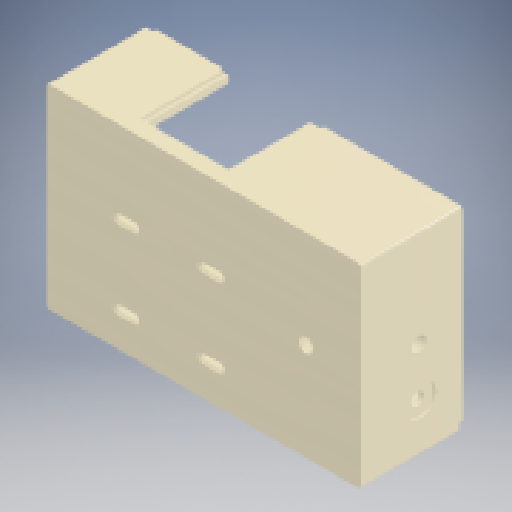
# Autodesk Inventor part: First_Stage_BoxBottom_Print
Saved by Autodesk Inventor 2025.2 (Build 292293000, 293)
## iProperties
Created: 2024-12-04
Part Number: First_Stage_BoxBottom_Print
Material: Generic
Document SubType Name: Modeling
Designer: Paul Linke
Density: 1 g/cm^3
Appearance: Light Beige
Author: Paul Linke
Autodesk Inventor part; units mm, degrees
ref_plane "YZ Plane" through (0, 0, 0) normal (1, 0, 0) x (0, 1, 0)
ref_plane "XZ Plane" through (0, 0, 0) normal (0, 1, 0) x (-1, 0, 0)
ref_plane "XY Plane" through (0, 0, 0) normal (0, 0, 1) x (1, 0, 0)
sketch "Sketch1" plane through (0, 0, 0) normal (0, 0, 1) x (1, 0, 0)
  line L0 (132.8531, -39.939) -> (132.8531, -33.679) projected
  line L1 (-45.1505, -5.78) -> (-45.1505, -12.04) projected
  circle A0 centre (47.6, -44.5) radius 1.45 projected
  circle A1 centre (0, -44.5) radius 1.45 projected
  circle A2 centre (0, 0) radius 1.45 projected
  circle A3 centre (47.5, 0) radius 1.45 projected
  line L2 (132.8531, -63.939) -> (-45.1505, -63.939)
  line L3 (-45.1505, 46.119) -> (132.8531, 46.119)
  line L4 (132.8531, 46.119) -> (132.8531, -63.939)
  line L5 (-45.1505, -63.939) -> (-45.1505, -12.04)
  line L6 (-45.1505, 46.119) -> (-45.1505, -5.78)
  line L7 (-45.1505, -12.04) -> (-45.1505, -5.78)
  line L8 (52.6, -44.5) -> (42.6, -44.5) construction
  line L9 (52.6, -43.05) -> (42.6, -43.05)
  line L10 (42.6, -45.95) -> (52.6, -45.95)
  arc A4 (52.6, -45.95) -> (52.6, -43.05) centre (52.6, -44.5) ccw
  arc A5 (42.6, -43.05) -> (42.6, -45.95) centre (42.6, -44.5) ccw
  line L11 (5, -44.5) -> (-5, -44.5) construction
  line L12 (5, -43.05) -> (-5, -43.05)
  line L13 (-5, -45.95) -> (5, -45.95)
  arc A6 (5, -45.95) -> (5, -43.05) centre (5, -44.5) ccw
  arc A7 (-5, -43.05) -> (-5, -45.95) centre (-5, -44.5) ccw
  line L14 (5, 0) -> (-5, 0) construction
  line L15 (5, 1.45) -> (-5, 1.45)
  line L16 (-5, -1.45) -> (5, -1.45)
  arc A8 (5, -1.45) -> (5, 1.45) centre (5, 0) ccw
  arc A9 (-5, 1.45) -> (-5, -1.45) centre (-5, 0) ccw
  line L17 (52.5, 0) -> (42.5, 0) construction
  line L18 (52.5, 1.45) -> (42.5, 1.45)
  line L19 (42.5, -1.45) -> (52.5, -1.45)
  arc A10 (52.5, -1.45) -> (52.5, 1.45) centre (52.5, 0) ccw
  arc A11 (42.5, 1.45) -> (42.5, -1.45) centre (42.5, 0) ccw
  point P0 (0, 0)
  dimension "d1" = 24
  dimension "d2" = 10
  dimension "d3" = 10
  dimension "d4" = 10
  dimension "d5" = 10
  constraints: 44 end point, 20 tangent, 16 point on circle, 8 centre point, 8 equal length, 4 midpoint, 2 collinear, 2 horizontal, 2 point on line, 1 vertical
  measures "d1" distance from line of L0.start L2
  measures "d2" distance of L8.end L8.start
  measures "d3" distance of L11.end L11.start
  measures "d4" distance of L17.end L17.start
  measures "d5" distance of L14.end L14.start
extrude "Extrusion1" add sketch "Sketch1" along normal blind 5
sketch "Sketch2" plane through (0, 0, 0) normal (0, 0, -1) x (-1, 0, 0)
  line L0 (41.1505, -59.939) -> (-128.8531, -59.939)
  line L1 (-128.8531, -59.939) -> (-128.8531, 42.119)
  line L2 (-128.8531, 42.119) -> (41.1505, 42.119)
  line L3 (41.1505, 42.119) -> (41.1505, -59.939)
  line L4 (45.1505, -63.939) -> (-132.8531, -63.939) projected
  line L5 (45.1505, 46.119) -> (45.1505, -63.939) projected
  line L6 (-132.8531, 46.119) -> (45.1505, 46.119) projected
  line L7 (-132.8531, -63.939) -> (-132.8531, 46.119) projected
  point P0 (0, 0)
  dimension "d8" = 4
  dimension "d9" = 4
  dimension "d10" = 4
  dimension "d11" = 4
  constraints: 8 end point, 2 parallel, 1 horizontal, 1 perpendicular
  measures "d8" distance between parallel lines of L0 L4
  measures "d9" distance between parallel lines of L5 L3
  measures "d10" distance between parallel lines of L2 L6
  measures "d11" distance between parallel lines of L7 L1
extrude "Extrusion2" add sketch "Sketch2" along normal blind 50
fillet "Fillet1" radius 2 4 edges at (-45.1505, 46.119, -22.5) (132.8531, 46.119, -22.5) (-45.1505, -63.939, -22.5) (132.8531, -63.939, -22.5)
fillet "Fillet2" radius 15 4 edges at (128.8531, -59.939, -25) (-41.1505, -59.939, -25) (-41.1505, 42.119, -25) (128.8531, 42.119, -25)
sketch "Sketch5" plane through (0, 0, -50) normal (0, 0, -1) x (-1, 0, 0)
  arc A0 (-132.8531, -61.939) -> (-130.8531, -63.939) centre (-130.8531, -61.939) ccw projected
  line L0 (-130.8531, -63.939) -> (43.1505, -63.939) projected
  arc A1 (43.1505, -63.939) -> (45.1505, -61.939) centre (43.1505, -61.939) ccw projected
  line L1 (45.1505, -61.939) -> (45.1505, 44.119) projected
  arc A2 (45.1505, 44.119) -> (43.1505, 46.119) centre (43.1505, 44.119) ccw projected
  line L2 (43.1505, 46.119) -> (-130.8531, 46.119) projected
  arc A3 (-130.8531, 46.119) -> (-132.8531, 44.119) centre (-130.8531, 44.119) ccw projected
  line L3 (-132.8531, 44.119) -> (-132.8531, -61.939) projected
  line L4 (26.1505, -59.939) -> (-113.8531, -59.939) projected
  arc A4 (-128.8531, -44.939) -> (-113.8531, -59.939) centre (-113.8531, -44.939) ccw projected
  line L5 (-128.8531, -44.939) -> (-128.8531, 27.119) projected
  arc A5 (-113.8531, 42.119) -> (-128.8531, 27.119) centre (-113.8531, 27.119) ccw projected
  line L6 (-113.8531, 42.119) -> (26.1505, 42.119) projected
  arc A6 (41.1505, 27.119) -> (26.1505, 42.119) centre (26.1505, 27.119) ccw projected
  line L7 (41.1505, 27.119) -> (41.1505, -44.939) projected
  arc A7 (26.1505, -59.939) -> (41.1505, -44.939) centre (26.1505, -44.939) ccw projected
  line L8 (43.1505, -61.939) -> (-130.8531, -61.939)
  line L9 (-130.8531, -61.939) -> (-130.8531, 44.119)
  line L10 (-130.8531, 44.119) -> (43.1505, 44.119)
  line L11 (43.1505, 44.119) -> (43.1505, -61.939)
  point P0 (0, 0)
  constraints: 8 end point, 2 parallel, 1 horizontal, 1 perpendicular
extrude "Extrusion3" add sketch "Sketch5" along normal blind 4 contours L8 L9 L10 L11
fillet "Fillet3" radius 2 4 edges at (-43.1505, 44.119, -52) (130.8531, 44.119, -52) (130.8531, -61.939, -52) (-43.1505, -61.939, -52)
sketch "Sketch12" plane through (-43.1505, -63.939, 5) normal (0, -1, 0) x (1, 0, 0)
  line L0 (157.0036, -5) -> (17, -5) projected
  line L1 (17, -59) -> (157.0036, -59) projected
  line L2 (91.972, -5) -> (41.972, -5)
  line L3 (41.972, -5) -> (41.972, -59)
  line L4 (41.972, -59) -> (91.972, -59)
  line L5 (91.972, -59) -> (91.972, -5)
  line L6 (91.972, -59) -> (41.972, -59)
  line L7 (91.972, -5) -> (41.972, -5)
  line L8 (91.972, -9) -> (41.972, -9)
  line L9 (41.972, -9) -> (41.972, -5)
  line L10 (41.972, -5) -> (91.972, -5)
  line L11 (91.972, -5) -> (91.972, -9)
  line L12 (95.972, -5) -> (95.972, -59)
  line L13 (37.972, -59) -> (37.972, -5)
  point P0 (43.1505, -5)
  point P1 (84.472, -31.9556)
  point P2 (49.472, -31.9556)
  point P3 (91.972, -32)
  point P4 (41.972, -32)
  dimension "d41" = 7.5
  dimension "d42" = 7.5
  dimension "d49" = 4
  constraints: 24 end point, 5 equal length, 3 perpendicular, 3 point on line, 2 horizontal, 2 midpoint, 2 vertical, 6 other
  measures "d41" horizontal distance of point (91.972, -32) point (84.472, -31.956)
  measures "d42" horizontal distance of point (41.972, -32) point (49.472, -31.956)
  measures "d49" distance between parallel lines of L0 L8
extrude "Extrusion9" cut sketch "Sketch12" against normal blind 150 contours L5 L1 L3 L8
sketch "Sketch13" plane through (113.8531, -59.939, 0) normal (0, 1, 0) x (1, 0, 0)
  line L0 (-140.0036, 54) -> (-115.0316, 54) projected
  line L1 (0, 0) -> (-140.0036, 0) projected
  line L2 (-119.0316, 54) -> (-61.0316, 54)
  line L3 (-61.0316, 54) -> (-61.0316, 0)
  line L4 (-61.0316, 0) -> (-119.0316, 0)
  line L5 (-119.0316, 0) -> (-119.0316, 54)
  line L6 (-115.0316, 4) -> (-115.0316, 54) projected
  line L7 (-65.0316, 54) -> (-65.0316, 4) projected
  point P0 (-113.8531, 0)
  point P1 (-75.0316, 0)
  point P2 (-125.0316, 0)
  point P3 (-65.0316, 4)
  point P4 (-119.0316, 0)
  dimension "d45" = 4
  dimension "d46" = 4
  constraints: 8 end point, 2 parallel, 2 point on line, 1 horizontal, 1 perpendicular, 2 other
extrude "Extrusion10" cut sketch "Sketch13" along normal blind 104.0581 and the other way blind 2
sketch "Sketch15" plane through (113.8531, -59.939, 0) normal (0, 1, 0) x (1, 0, 0)
  line L0 (-61.0316, 50) -> (-61.0316, 54) projected
  line L1 (-61.0316, 50) -> (-61.0316, 0) projected
  line L2 (-61.0316, 0) -> (-119.0316, 0) projected
  line L3 (-119.0316, 0) -> (-119.0316, 50) projected
  line L4 (-119.0316, 54) -> (-119.0316, 50) projected
  line L5 (-114.9316, 4.1) -> (-114.9316, 50)
  line L6 (-115.0316, 50) -> (-115.0316, 4) projected
  line L7 (-115.0316, 4) -> (-65.0316, 4) projected
  line L8 (-65.0316, 4) -> (-65.0316, 50) projected
  line L9 (-65.0316, 50) -> (-65.0316, 4) projected
  line L10 (0, 0) -> (-61.0316, 0) projected
  line L11 (-65.0316, 50) -> (-57.0316, 50)
  line L12 (-57.0316, 50) -> (-57.0316, 0)
  line L13 (-57.0316, 0) -> (-65.0316, 0)
  line L14 (-65.0316, 0) -> (-65.0316, 50)
  line L15 (-115.0316, 50) -> (-123.0316, 50)
  line L16 (-123.0316, 50) -> (-123.0316, 0)
  line L17 (-123.0316, 0) -> (-115.0316, 0)
  line L18 (-115.0316, 0) -> (-115.0316, 50)
  line L19 (-65.0316, 4) -> (-115.0316, 4)
  line L20 (-115.0316, 4) -> (-115.0316, 0)
  line L21 (-115.0316, 0) -> (-65.0316, 0)
  line L22 (-65.0316, 0) -> (-65.0316, 4)
  line L23 (-57.0316, 50) -> (-65.0316, 50)
  line L24 (-65.0316, 50) -> (-65.0316, 54)
  line L25 (-65.0316, 54) -> (-57.0316, 54)
  line L26 (-57.0316, 54) -> (-57.0316, 50)
  line L27 (-115.0316, 50) -> (-119.0316, 50) projected
  line L28 (-140.0036, 54) -> (-119.0316, 54) projected
  line L29 (-115.0316, 50) -> (-123.0316, 50)
  line L30 (-123.0316, 50) -> (-123.0316, 54)
  line L31 (-123.0316, 54) -> (-115.0316, 54)
  line L32 (-115.0316, 54) -> (-115.0316, 50)
  point P0 (-119.0316, 0)
  dimension "d124" = 8
  dimension "d125" = 8
  constraints: 42 end point, 10 parallel, 5 horizontal, 5 perpendicular, 3 point on line, 1 vertical, 2 other
  measures "d124" distance of L12.end L13.end
  measures "d125" distance of L17.end L16.end
extrude "Extrusion12" add sketch "Sketch15" along normal blind 4
sketch "Sketch17" plane through (-45.1505, -61.939, 5) normal (-1, 0, 0) x (0, 0, 1)
  line L0 (-55, -2) -> (0, -2) projected
  line L1 (0, 108.058) -> (-55, 108.058) projected
  line L2 (0, 106.058) -> (-55, 106.058) projected
  circle A0 centre (-32.44, 53.029) radius 2.305
  circle A1 centre (-32.44, 53.029) radius 3.5
  point P0 (-5, 61.939)
  dimension "d114" = 7
  constraints: 2 centre point, 1 coincident, 2 other
  measures "d114" diameter of A1
extrude "Extrusion14" cut sketch "Sketch17" against normal blind 10 contours A0 | A1
sketch "Sketch18" plane through (-45.1505, -61.939, 5) normal (-1, 0, 0) x (0, 0, 1)
  circle A0 centre (-32.44, 53.029) radius 2.555
  circle A1 centre (-32.44, 53.029) radius 3.5 projected
  circle A2 centre (-32.44, 53.029) radius 9
  point P0 (-5, 61.939)
  dimension "d115" = 18
  constraints: 2 centre point, 1 coincident, 2 other
  measures "d115" diameter of A2
extrude "Extrusion15" cut sketch "Sketch18" against normal blind 1.3 contours A0 | A1 | A2
sketch "Sketch19" plane through (132.8531, -61.939, -50) normal (1, 0, 0) x (0, 0, -1)
  circle A0 centre (-21.8645, 25.1387) radius 2.425
  circle A1 centre (-21.8645, 25.1387) radius 3.5
  point P0 (-50, 61.939)
  dimension "d116" = 7
  constraints: 2 centre point, 1 coincident, 2 other
  measures "d116" diameter of A1
extrude "Extrusion16" cut sketch "Sketch19" against normal blind 10 contours A0 | A1
sketch "Sketch20" plane through (132.8531, -61.939, -50) normal (1, 0, 0) x (0, 0, -1)
  circle A0 centre (-21.8645, 25.1387) radius 2.555
  circle A1 centre (-21.8645, 25.1387) radius 9
  point P0 (-50, 61.939)
  dimension "d117" = 18
  constraints: 2 centre point, 1 coincident, 2 other
  measures "d117" diameter of A1
extrude "Extrusion17" cut sketch "Sketch20" against normal blind 1.3 contours A0 | A1
sketch "Sketch23" plane through (0, 0, 0) normal (0, 0, -1) x (-1, 0, 0)
  line L0 (9.1785, -59.939) -> (26.1505, -59.939) projected
  arc A0 (26.1505, -59.939) -> (41.1505, -44.939) centre (26.1505, -44.939) ccw projected
  line L1 (41.1505, -44.939) -> (41.1505, 27.119) projected
  arc A1 (41.1505, 27.119) -> (26.1505, 42.119) centre (26.1505, 27.119) ccw projected
  line L2 (26.1505, 42.119) -> (5.1785, 42.119) projected
  arc A2 (-113.8531, 42.119) -> (-128.8531, 27.119) centre (-113.8531, 27.119) ccw projected
  line L3 (-128.8531, 27.119) -> (-128.8531, -44.939) projected
  arc A3 (-128.8531, -44.939) -> (-113.8531, -59.939) centre (-113.8531, -44.939) ccw projected
  line L4 (-113.8531, -59.939) -> (-56.8215, -59.939) projected
  arc A4 (-52.6, -43.05) -> (-52.6, -45.95) centre (-52.6, -44.5) ccw projected
  line L5 (-42.6, -43.05) -> (-52.6, -43.05) projected
  arc A5 (-42.6, -45.95) -> (-42.6, -43.05) centre (-42.6, -44.5) ccw projected
  line L6 (-52.6, -45.95) -> (-42.6, -45.95) projected
  arc A6 (-5, -43.05) -> (-5, -45.95) centre (-5, -44.5) ccw projected
  line L7 (5, -43.05) -> (-5, -43.05) projected
  arc A7 (5, -45.95) -> (5, -43.05) centre (5, -44.5) ccw projected
  line L8 (-5, -45.95) -> (5, -45.95) projected
  arc A8 (-5, 1.45) -> (-5, -1.45) centre (-5, 0) ccw projected
  line L9 (5, 1.45) -> (-5, 1.45) projected
  arc A9 (5, -1.45) -> (5, 1.45) centre (5, 0) ccw projected
  line L10 (-5, -1.45) -> (5, -1.45) projected
  arc A10 (-52.5, 1.45) -> (-52.5, -1.45) centre (-52.5, 0) ccw projected
  line L11 (-42.5, 1.45) -> (-52.5, 1.45) projected
  arc A11 (-42.5, -1.45) -> (-42.5, 1.45) centre (-42.5, 0) ccw projected
  line L12 (-52.5, -1.45) -> (-42.5, -1.45) projected
  line L13 (-73.8531, 6.09) -> (-128.8531, 6.09)
  line L14 (-128.8531, 6.09) -> (-128.8531, -23.91)
  line L15 (-128.8531, -23.91) -> (-73.8531, -23.91)
  line L16 (-73.8531, -23.91) -> (-73.8531, 6.09)
  line L17 (-128.8531, -44.939) -> (-128.8531, 27.119) projected
  line L18 (43.1505, 46.119) -> (-130.8531, 46.119) projected
  line L19 (-107.0925, 46.119) -> (-107.0925, 6.09) construction
  line L20 (-106.4911, -23.91) -> (-106.4911, -63.939) construction
  line L21 (43.1505, -63.939) -> (-130.8531, -63.939) projected
  line L22 (5.1785, 44.1191) -> (5.1785, 42.119) projected
  line L23 (-52.8215, 42.119) -> (-52.8215, 44.1191) projected
  line L24 (-52.8215, -61.939) -> (5.1785, -61.939) projected
  line L25 (5.1785, 44.1191) -> (-52.8215, 44.1191) projected
  line L26 (-52.8215, 42.119) -> (-113.8531, 42.119) projected
  line L27 (-52.8215, -61.939) -> (-52.8215, -59.939) projected
  line L28 (5.1785, -59.939) -> (5.1785, -61.939) projected
  line L29 (-56.8215, -59.939) -> (-56.8215, -55.939) projected
  line L30 (-56.8215, -55.939) -> (9.1785, -55.939) projected
  line L31 (9.1785, -55.939) -> (9.1785, -59.939) projected
  line L32 (5.1785, -59.939) -> (-52.8215, -59.939) projected
  point P0 (0, 0)
  point P1 (-128.8531, 6.09)
  point P2 (-128.8531, -23.91)
  dimension "d78" = 55
  dimension "d79" = 30
  constraints: 12 end point, 4 parallel, 4 point on line, 2 perpendicular, 1 collinear, 1 horizontal
  measures "d78" distance of L14.end L15.end
  measures "d79" distance between parallel lines of L15 L13
extrude "Extrusion19" add sketch "Sketch23" along normal blind 54 contours L3 L13 L16 L15
chamfer "Chamfer1" distance 54 angle 45 1 edges at (73.8531, -8.91, -54)
sketch "Sketch24" plane through (0, 0, 0) normal (0, 0, -1) x (-1, 0, 0)
  line L0 (-128.8531, 27.119) -> (-128.8531, 6.09) projected
  arc A0 (-128.8531, -44.939) -> (-113.8531, -59.939) centre (-113.8531, -44.939) ccw projected
  line L1 (9.1785, -59.939) -> (26.1505, -59.939) projected
  line L2 (-113.8531, -59.939) -> (-56.8215, -59.939) projected
  arc A1 (26.1505, -59.939) -> (41.1505, -44.939) centre (26.1505, -44.939) ccw projected
  line L3 (41.1505, -44.939) -> (41.1505, 27.119) projected
  arc A2 (41.1505, 27.119) -> (26.1505, 42.119) centre (26.1505, 27.119) ccw projected
  line L4 (26.1505, 42.119) -> (5.1785, 42.119) projected
  arc A3 (-113.8531, 42.119) -> (-128.8531, 27.119) centre (-113.8531, 27.119) ccw projected
  line L5 (-128.8531, -23.91) -> (-128.8531, -44.939) projected
  arc A4 (-52.6, -43.05) -> (-52.6, -45.95) centre (-52.6, -44.5) ccw projected
  line L6 (-42.6, -43.05) -> (-52.6, -43.05) projected
  arc A5 (-42.6, -45.95) -> (-42.6, -43.05) centre (-42.6, -44.5) ccw projected
  line L7 (-52.6, -45.95) -> (-42.6, -45.95) projected
  arc A6 (-5, -43.05) -> (-5, -45.95) centre (-5, -44.5) ccw projected
  line L8 (5, -43.05) -> (-5, -43.05) projected
  arc A7 (5, -45.95) -> (5, -43.05) centre (5, -44.5) ccw projected
  line L9 (-5, -45.95) -> (5, -45.95) projected
  arc A8 (-5, 1.45) -> (-5, -1.45) centre (-5, 0) ccw projected
  line L10 (5, 1.45) -> (-5, 1.45) projected
  arc A9 (5, -1.45) -> (5, 1.45) centre (5, 0) ccw projected
  line L11 (-5, -1.45) -> (5, -1.45) projected
  arc A10 (-52.5, 1.45) -> (-52.5, -1.45) centre (-52.5, 0) ccw projected
  line L12 (-42.5, 1.45) -> (-52.5, 1.45) projected
  arc A11 (-42.5, -1.45) -> (-42.5, 1.45) centre (-42.5, 0) ccw projected
  line L13 (-52.5, -1.45) -> (-42.5, -1.45) projected
  line L14 (-113.8531, 42.119) -> (26.1505, 42.119) projected
  line L15 (22.6785, 42.119) -> (17.6785, 42.119)
  line L16 (17.6785, 42.119) -> (17.6785, -59.939)
  line L17 (17.6785, -59.939) -> (22.6785, -59.939)
  line L18 (-60.3215, 42.119) -> (-65.3215, 42.119)
  line L19 (-65.3215, -59.939) -> (-60.3215, -59.939)
  line L20 (-60.3215, -59.939) -> (-60.3215, 42.119)
  line L21 (11.6785, -59.939) -> (11.6785, -55.439) projected
  line L22 (41.1505, 27.119) -> (41.1505, -44.939) projected
  line L23 (41.1505, -6.41) -> (22.6785, -6.41)
  line L24 (22.6785, -11.41) -> (41.1505, -11.41)
  line L25 (41.1505, -11.41) -> (41.1505, -6.41)
  line L26 (22.6785, -59.939) -> (22.6785, -11.41)
  line L27 (22.6785, -6.41) -> (22.6785, 42.119)
  line L28 (-65.3215, -6.41) -> (-110.0821, -6.41)
  line L29 (-110.0821, -6.41) -> (-110.0821, -11.41)
  line L30 (-110.0821, -11.41) -> (-65.3215, -11.41)
  line L31 (-65.3215, 42.119) -> (-65.3215, -6.41)
  line L32 (-65.3215, -11.41) -> (-65.3215, -59.939)
  line L33 (-128.8531, 6.09) -> (-73.8531, 6.09) projected
  line L34 (-73.8531, 6.09) -> (-73.8531, -23.91) projected
  line L35 (-73.8531, -23.91) -> (-128.8531, -23.91) projected
  line L36 (5.1785, 44.1191) -> (5.1785, 42.119) projected
  line L37 (-52.8215, 42.119) -> (-52.8215, 44.1191) projected
  line L38 (-52.8215, -61.939) -> (5.1785, -61.939) projected
  line L39 (5.1785, 44.1191) -> (-52.8215, 44.1191) projected
  line L40 (-52.8215, 42.119) -> (-113.8531, 42.119) projected
  line L41 (-52.8215, -61.939) -> (-52.8215, -59.939) projected
  line L42 (5.1785, -59.939) -> (5.1785, -61.939) projected
  line L43 (-56.8215, -59.939) -> (-56.8215, -55.939) projected
  line L44 (-56.8215, -55.939) -> (9.1785, -55.939) projected
  line L45 (9.1785, -55.939) -> (9.1785, -59.939) projected
  line L46 (5.1785, -59.939) -> (-52.8215, -59.939) projected
  point P0 (0, 0)
  point P1 (9.1785, -55.439)
  point P2 (11.6785, -56.9946)
  point P3 (-60.3215, -59.939)
  point P4 (-62.8215, 42.119)
  point P5 (-67.8215, 42.119)
  point P6 (22.6785, 42.119)
  point P7 (17.6785, 42.119)
  point P8 (22.6785, -59.939)
  point P9 (-52.8215, 42.119)
  point P10 (5.1785, 42.119)
  point P11 (-73.8531, -6.41)
  point P12 (-73.8531, -11.41)
  point P13 (-65.3215, 42.119)
  point P14 (17.6785, -59.939)
  dimension "d94" = 6
  dimension "d98" = 5
  dimension "d99" = 5
  dimension "d100" = 5
  constraints: 32 end point, 8 parallel, 5 collinear, 5 point on line, 4 horizontal, 4 perpendicular, 2 other
  measures "d94" distance from line of point (11.679, -56.995) L16
  measures "d98" distance between parallel lines of L24 L23
  measures "d99" distance between parallel lines of L16 L26
  measures "d100" distance between parallel lines of L32 L20
extrude "Extrusion20" add sketch "Sketch24" along normal blind 10 contours L14 L20 L2 L32 L30 L34 L28 L31 | L34 L30 L29 L28 | L4 L27 L23 L3 L24 L26 L1 L16
chamfer "Chamfer2" distance 7 angle 45 6 edges at (-41.1505, -8.91, -10) (-20.1785, -59.939, -10) (62.8215, -59.939, -10) (83.8526, -8.91, -10) (62.8215, 42.119, -10) (-20.1785, 42.119, -10)
sketch "Sketch25" plane through (113.8531, 42.119, -54) normal (0, -1, 0) x (1, 0, 0)
  line L0 (-115.0316, 50) -> (-115.0316, 0) projected
  line L1 (-119.0316, 4) -> (-119.0316, 54) projected
  line L2 (-119.0316, 4) -> (-119.0316, 0) projected
  line L3 (-61.1316, 0) -> (-118.9316, 0)
  line L4 (-65.0316, 4) -> (-65.0316, 50) projected
  line L5 (-65.0316, 0) -> (-65.0316, 50) projected
  line L6 (-61.0316, 0) -> (-61.0316, 4) projected
  line L7 (-61.0316, 54) -> (-61.0316, 4) projected
  line L8 (-65.0316, 50) -> (-115.0316, 50) projected
  line L9 (-119.0316, 54) -> (-61.0316, 54) projected
  line L10 (-57.0316, 54) -> (-123.0316, 54) projected
  line L11 (-115.0316, 0) -> (-123.0316, 0)
  line L12 (-123.0316, 0) -> (-123.0316, 54)
  line L13 (-123.0316, 54) -> (-115.0316, 54)
  line L14 (-115.0316, 54) -> (-115.0316, 0)
  line L15 (-65.0316, 0) -> (-57.0316, 0)
  line L16 (-57.0316, 0) -> (-57.0316, 54)
  line L17 (-57.0316, 54) -> (-65.0316, 54)
  line L18 (-65.0316, 54) -> (-65.0316, 0)
  point P0 (-124.5616, -37.6811)
  point P1 (-66.5616, 16.3189)
  point P2 (-70.5616, 12.3189)
  point P3 (-120.5616, 12.3189)
  point P4 (-61.1316, 0)
  point P5 (-57.0316, 54)
  dimension "d126" = 8
  constraints: 18 end point, 4 parallel, 3 horizontal, 2 perpendicular, 1 point on line, 2 other
  measures "d126" distance of L17.end L16.end
extrude "Extrusion21" add sketch "Sketch25" along normal blind 4 contours L14 L9 L18 L8 | L0 L3 L11 L2 L1 L9 L14 | L18 L9 L7 L6 L15 L3 L5 L4 | L1 L2 L11 L12 L10 | L10 L16 L15 L6 L7
sketch "Sketch26" plane through (0, 0, 0) normal (0, 0, -1) x (-1, 0, 0)
  arc A0 (-5, -43.05) -> (-5, -45.95) centre (-5, -44.5) ccw projected
  line L0 (5, -43.05) -> (-5, -43.05) projected
  arc A1 (5, -45.95) -> (5, -43.05) centre (5, -44.5) ccw projected
  line L1 (-5, -45.95) -> (5, -45.95) projected
  arc A2 (-42.5, -1.45) -> (-42.5, 1.45) centre (-42.5, 0) ccw projected
  arc A3 (-52.5, 1.45) -> (-52.5, -1.45) centre (-52.5, 0) ccw projected
  line L2 (-42.5, 1.45) -> (-52.5, 1.45) projected
  line L3 (-52.5, -1.45) -> (-42.5, -1.45) projected
  line L4 (5, -44.5) -> (0, -44.5)
  line L5 (0, -44.5) -> (-5, -44.5)
  circle A4 centre (0, -44.5) radius 1.45
  line L6 (-47.5, 0) -> (-52.5, 0)
  line L7 (-42.5, 0) -> (-47.5, 0)
  circle A5 centre (-47.5, 0) radius 1.45
  point P0 (0, 0)
  constraints: 8 end point, 4 collinear, 2 centre point, 2 coincident, 1 horizontal
sketch "Sketch27" plane through (0, 0, -54) normal (0, 0, -1) x (-1, 0, 0)
  line L0 (9.1785, 42.119) -> (26.1505, 42.119) projected
  arc A0 (41.1505, 27.119) -> (26.1505, 42.119) centre (26.1505, 27.119) ccw projected
  line L1 (41.1505, 27.119) -> (41.1505, -44.939) projected
  arc A1 (26.1505, -59.939) -> (41.1505, -44.939) centre (26.1505, -44.939) ccw projected
  line L2 (26.1505, -59.939) -> (9.1785, -59.939) projected
  line L3 (-56.8215, -59.939) -> (-113.8531, -59.939) projected
  arc A2 (-128.8531, -44.939) -> (-113.8531, -59.939) centre (-113.8531, -44.939) ccw projected
  line L4 (-128.8531, -44.939) -> (-128.8531, -23.91) projected
  line L5 (-128.8531, -23.91) -> (-127.8531, -23.91) projected
  line L6 (-127.8531, 6.09) -> (-127.8531, -23.91) projected
  line L7 (-127.8531, 6.09) -> (-128.8531, 6.09) projected
  line L8 (-128.8531, 6.09) -> (-128.8531, 27.119) projected
  arc A3 (-113.8531, 42.119) -> (-128.8531, 27.119) centre (-113.8531, 27.119) ccw projected
  line L9 (-113.8531, 42.119) -> (-56.8215, 42.119) projected
  line L10 (-52.8215, 42.119) -> (-52.8215, 44.119) projected
  line L11 (-52.8215, 44.119) -> (-128.8531, 44.119) projected
  arc A4 (-128.8531, 44.119) -> (-130.8531, 42.119) centre (-128.8531, 42.119) ccw projected
  line L12 (-130.8531, 42.119) -> (-130.8531, -59.939) projected
  arc A5 (-130.8531, -59.939) -> (-128.8531, -61.939) centre (-128.8531, -59.939) ccw projected
  line L13 (-128.8531, -61.939) -> (-52.8215, -61.939) projected
  line L14 (-52.8215, -61.939) -> (-52.8215, -59.939) projected
  line L15 (5.1785, -59.939) -> (5.1785, -61.939) projected
  line L16 (5.1785, -61.939) -> (41.1505, -61.939) projected
  arc A6 (41.1505, -61.939) -> (43.1505, -59.939) centre (41.1505, -59.939) ccw projected
  line L17 (43.1505, -59.939) -> (43.1505, 42.119) projected
  arc A7 (43.1505, 42.119) -> (41.1505, 44.119) centre (41.1505, 42.119) ccw projected
  line L18 (41.1505, 44.119) -> (5.1785, 44.119) projected
  line L19 (5.1785, 44.119) -> (5.1785, 42.119) projected
  line L20 (-130.2673, 43.5332) -> (-127.3635, 40.6294) construction
  line L21 (-127.3635, 40.6294) -> (-124.4597, 37.7256) construction
  circle A8 centre (-127.3635, 40.6294) radius 2
  line L22 (-130.2673, -61.3532) -> (-127.3635, -58.4494) construction
  line L23 (-127.3635, -58.4494) -> (-124.4597, -55.5456) construction
  circle A9 centre (-127.3635, -58.4494) radius 2
  line L24 (42.5647, -61.3532) -> (39.6609, -58.4494) construction
  line L25 (39.6609, -58.4494) -> (36.7571, -55.5456) construction
  circle A10 centre (39.6609, -58.4494) radius 2
  line L26 (36.7571, 37.7256) -> (39.6609, 40.6294) construction
  line L27 (39.6609, 40.6294) -> (42.5647, 43.5332) construction
  circle A11 centre (39.6609, 40.6294) radius 2
  line L28 (-52.8215, -59.939) -> (-48.8215, -59.939) projected
  line L29 (-48.8215, -59.939) -> (-48.8215, -55.939) projected
  line L30 (-56.8215, -55.939) -> (-48.8215, -55.939) projected
  line L31 (-56.8215, -59.939) -> (-56.8215, -55.939) projected
  line L32 (9.1785, -59.939) -> (9.1785, -55.939) projected
  line L33 (1.1785, -55.939) -> (9.1785, -55.939) projected
  line L34 (1.1785, -59.939) -> (1.1785, -55.939) projected
  line L35 (1.1785, -59.939) -> (5.1785, -59.939) projected
  line L36 (5.1785, 42.119) -> (1.1785, 42.119) projected
  line L37 (1.1785, 42.119) -> (1.1785, 38.119) projected
  line L38 (9.1785, 38.119) -> (1.1785, 38.119) projected
  line L39 (9.1785, 42.119) -> (9.1785, 38.119) projected
  line L40 (-56.8215, 42.119) -> (-56.8215, 38.119) projected
  line L41 (-48.8215, 38.119) -> (-56.8215, 38.119) projected
  line L42 (-48.8215, 42.119) -> (-48.8215, 38.119) projected
  line L43 (-48.8215, 42.119) -> (-52.8215, 42.119) projected
  point P0 (0, 0)
  dimension "d118" = 4
  dimension "d119" = 4
  dimension "d120" = 4
  dimension "d121" = 4
  constraints: 16 end point, 8 point on circle, 4 centre point, 4 collinear, 3 coincident, 1 point on line
  measures "d118" diameter of A8
  measures "d119" diameter of A9
  measures "d120" diameter of A10
  measures "d121" diameter of A11
extrude "Extrusion22" cut sketch "Sketch27" against normal blind 7 contours A8 | A9 | A10 | A11
sketch "Sketch28" plane through (132.8531, -61.939, -50) normal (1, 0, 0) x (0, 0, -1)
  line L0 (4, 68.029) -> (-50, 68.029) projected
  line L1 (-50, 38.029) -> (4, 38.029) projected
  line L2 (0, 106.058) -> (0, 0) projected
  line L3 (-50, 50.529) -> (-50, 38.029) projected
  line L4 (-50, 104.058) -> (-50, 2) projected
  line L5 (9, 106.058) -> (9, 0)
  circle A0 centre (-22.56, 53.029) radius 2.921
  circle A1 centre (-22.56, 53.029) radius 3.5 projected
  circle A2 centre (-22.56, 53.029) radius 4
  point P0 (-50, 61.939)
  dimension "d127" = 8
  constraints: 2 centre point, 2 end point, 1 coincident, 1 vertical, 4 other
  measures "d127" diameter of A2
extrude "Extrusion23" cut sketch "Sketch28" against normal blind 15 contours A0 | A1 | A2
sketch "Sketch29" plane through (0, 0, 5) normal (0, 0, 1) x (1, 0, 0)
  line L0 (73.8531, 6.09) -> (73.8531, -6.41) projected
  line L1 (73.8531, -11.41) -> (73.8531, -23.91) projected
  line L2 (73.8531, -23.91) -> (128.8531, -23.91) projected
  line L3 (128.8531, 6.09) -> (73.8531, 6.09) projected
  line L4 (128.8531, -23.91) -> (128.8531, -44.939) projected
  line L5 (128.8531, 27.119) -> (128.8531, 6.09) projected
  line L6 (132.8531, -61.939) -> (132.8531, 44.119) projected
  line L7 (73.8531, -23.91) -> (128.8531, 6.09) construction
  line L8 (128.8531, -23.91) -> (73.8531, 6.09) construction
  circle A0 centre (101.3531, -8.91) radius 4
  point P0 (0, 0)
  dimension "d130" = 8
  constraints: 4 end point, 1 centre point, 1 midpoint
  measures "d130" diameter of A0
extrude "Extrusion24" cut sketch "Sketch29" against normal blind 15
sketch "Sketch30" plane through (-43.1505, -63.939, 5) normal (0, -1, 0) x (1, 0, 0)
  line L0 (25.472, -22) -> (25.472, -5) projected
  line L1 (25.472, -22) -> (20.472, -22) projected
  line L2 (20.472, -5) -> (20.472, -22) projected
  line L3 (41.972, -55) -> (0, -55) projected
  line L4 (22.972, -7.9954) -> (22.972, -57.7233) construction
  circle A0 centre (22.972, -44.0236) radius 3.5
  point P0 (43.1505, -5)
  dimension "d133" = 7
  constraints: 2 end point, 1 centre point, 1 perpendicular, 1 point on line
  measures "d133" diameter of A0
extrude "Extrusion25" cut sketch "Sketch30" against normal blind 10
sketch "Sketch31" plane through (-43.1505, -63.939, 5) normal (0, -1, 0) x (1, 0, 0)
  circle A0 centre (22.972, -44.0236) radius 3.5 projected
  circle A1 centre (22.972, -44.0236) radius 9
  point P0 (43.1505, -5)
  dimension "d136" = 18
  constraints: 1 centre point, 1 coincident
  measures "d136" diameter of A1
extrude "Extrusion26" cut sketch "Sketch31" against normal blind 1.3 contours A0 | A1
sketch "Sketch32" plane through (-26.1505, -59.939, 0) normal (0, 1, 0) x (1, 0, 0)
  circle A0 centre (5.972, 39.0236) radius 3.5 projected
  circle A1 centre (5.972, 39.0236) radius 9 projected
  point P0 (26.1505, 0)
extrude "Extrusion27" cut sketch "Sketch32" along normal mid plane 2 contours A0 | A1
chamfer "Chamfer4" distance 1.3 angle 45 16 edges at (0, -1.45, 5) (-6.45, 0, 5) (0, 1.45, 5) (6.45, 0, 5) (47.5, -1.45, 5) (41.05, 0, 5) (47.5, 1.45, 5) (53.95, 0, 5) (47.6, -45.95, 5) (41.15, -44.5, 5) (47.6, -43.05, 5) (54.05, -44.5, 5) (0, -45.95, 5) (-6.45, -44.5, 5) (0, -43.05, 5) (6.45, -44.5, 5)
body "Solid1"
